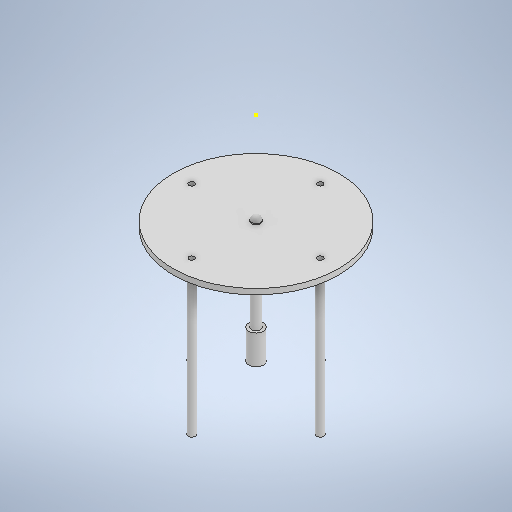
# Autodesk Inventor part: tarcza
Saved by Autodesk Inventor 2025 (Build 290162000, 162)
## iProperties
Created: 2024-12-31
Part Number: tarcza
Material: Ogólny
Document SubType Name: Modeling
Designer: Laptop
Density: 1 g/cm^3
Appearance: Domyślna
Author: Laptop
Autodesk Inventor part; units mm, degrees
ref_plane "YZ Plane" through (0, 0, 0) normal (1, 0, 0) x (0, 1, 0)
ref_plane "XZ Plane" through (0, 0, 0) normal (0, 1, 0) x (-1, 0, 0)
ref_plane "XY Plane" through (0, 0, 0) normal (0, 0, 1) x (1, 0, 0)
sketch "Szkic1" plane through (0, 0, 0) normal (0, 1, 0) x (-1, 0, 0)
  circle A0 centre (0, 0) radius 45
  circle A1 centre (35, 0) radius 1.5
  circle A2 centre (-35, 0) radius 1.5
  circle A3 centre (0, 35) radius 1.5
  circle A4 centre (0, -35) radius 1.5
  dimension "d0" = 90
  dimension "d30" = 3
  dimension "d31" = 3
  dimension "d32" = 3
  dimension "d33" = 3
  constraints: 5 centre point, 1 coincident
  measures "d0" diameter of A0
  measures "d30" diameter of A1
  measures "d31" diameter of A2
  measures "d32" diameter of A3
  measures "d33" diameter of A4
extrude "Wyciągnięcie proste1" add sketch "Szkic1" along normal blind 3 contours A0 | A1 | A2 | A3 | A4
sketch "Szkic2" plane through (0, 3, 0) normal (0, 1, 0) x (1, 0, 0)
  point P0 (0, 0)
extrude "Wyciągnięcie proste3" [suppressed]
sketch "Szkic3" plane through (0, 3, 0) normal (0, 1, 0) x (1, 0, 0)
  circle A0 centre (0, 0) radius 2.5
  dimension "d15" = 5
  constraints: 1 centre point, 1 coincident
  measures "d15" diameter of A0
extrude "Wyciągnięcie proste4" add sketch "Szkic3" along normal mid plane 100
sketch "Szkic4" plane through (0, 0, 0) normal (0, -1, 0) x (1, 0, 0)
  circle A0 centre (0, 0) radius 2.5 projected
  circle A1 centre (0, 0) radius 2
  dimension "d19" = 4
  constraints: 1 centre point, 1 coincident
  measures "d19" diameter of A1
extrude "Wyciągnięcie proste5" cut sketch "Szkic4" against normal blind 2 contours A1
sketch "Szkic8" plane through (0, 2, 0) normal (0, -1, 0) x (1, 0, 0)
  point P0 (0, 0)
sketch "Szkic9" plane through (0, -47, 0) normal (0, -1, 0) x (1, 0, 0)
  circle A0 centre (0, 0) radius 2 projected
  circle A1 centre (0, 0) radius 4
  dimension "d22" = 8
  constraints: 1 centre point, 1 coincident
  measures "d22" diameter of A1
extrude "Wyciągnięcie proste6" add sketch "Szkic9" along normal blind 16 contours A0 | A1
sketch "Szkic12" plane through (0, -63, 0) normal (0, -1, 0) x (1, 0, 0)
  circle A0 centre (0, 0) radius 2.5 projected
  circle A1 centre (0, 0) radius 2.5
  constraints: 1 centre point, 1 coincident
extrude "Wyciągnięcie proste7" cut sketch "Szkic12" against normal blind 10
sketch "Szkic13" plane through (0, 53, 0) normal (0, 1, 0) x (1, 0, 0)
  point P0 (0, 0)
sketch "Szkic14" plane through (0, 53, 0) normal (0, 1, 0) x (1, 0, 0)
  circle A0 centre (0, 0) radius 4 projected
  circle A1 centre (0, 0) radius 4
  constraints: 1 centre point, 1 coincident
extrude "Wyciągnięcie proste8" cut sketch "Szkic14" against normal blind 47
fillet "Zaokrąglenie2" radius 2.5 1 edges at (-2.5, 6, 0)
sketch "Szkic17" plane through (0, 3, 0) normal (0, 1, 0) x (1, 0, 0)
  circle A0 centre (-35, 0) radius 1.5
  circle A1 centre (0, 35) radius 1.5
  circle A2 centre (0, -35) radius 1.5
  circle A3 centre (35, 0) radius 1.5
  point P0 (0, 0)
  dimension "d34" = 3
  dimension "d35" = 3
  dimension "d36" = 3
  dimension "d37" = 3
  constraints: 4 centre point
  measures "d34" diameter of A0
  measures "d35" diameter of A1
  measures "d36" diameter of A2
  measures "d37" diameter of A3
extrude "Wyciągnięcie proste9" cut sketch "Szkic17" against normal blind 47
sketch "Szkic18" plane through (0, 0, 0) normal (0, -1, 0) x (1, 0, 0)
  circle A0 centre (0, 35) radius 1.5 projected
  circle A1 centre (0, 35) radius 2
  circle A2 centre (-35, 0) radius 1.5 projected
  circle A3 centre (-35, 0) radius 2
  circle A4 centre (0, -35) radius 1.5 projected
  circle A5 centre (0, -35) radius 2
  circle A6 centre (35, 0) radius 1.5 projected
  circle A7 centre (35, 0) radius 1.5
  circle A8 centre (35, 0) radius 2
  point P0 (0, 0)
  dimension "d40" = 4
  dimension "d41" = 4
  dimension "d42" = 4
  dimension "d43" = 3
  dimension "d44" = 4
  constraints: 5 centre point, 5 coincident
  measures "d40" diameter of A1
  measures "d41" diameter of A3
  measures "d42" diameter of A5
  measures "d43" diameter of A7
  measures "d44" diameter of A8
extrude "Wyciągnięcie proste10" add sketch "Szkic18" along normal blind 80
